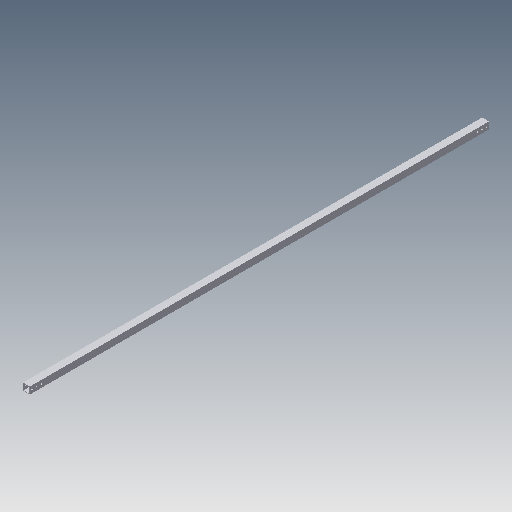
# Autodesk Inventor part: □15
Saved by Autodesk Inventor 2019.4 (Build 234330000, 330)
## iProperties
Created: 2018-08-09
Part Number: □15
Material: 一般
Document SubType Name: Modeling
Designer: Owner
Density: 1 g/cm^3
Appearance: 既定
Mass: 44.7093 g
Surface Area: 896.475 cm^2
Volume: 44.7093 cm^3
Author: Owner
Autodesk Inventor part; units mm, degrees
ref_plane "YZ Plane" through (0, 0, 0) normal (1, 0, 0) x (0, 1, 0)
ref_plane "XZ Plane" through (0, 0, 0) normal (0, 1, 0) x (-1, 0, 0)
ref_plane "XY Plane" through (0, 0, 0) normal (0, 0, 1) x (1, 0, 0)
sketch "スケッチ1" plane through (0, 0, 0) normal (0, 0, 1) x (1, 0, 0)
  line L0 (7.5, 7.5) -> (-7.5, 7.5)
  line L1 (-7.5, 7.5) -> (-7.5, -7.5)
  line L2 (-7.5, -7.5) -> (7.5, -7.5)
  line L3 (7.5, -7.5) -> (7.5, 7.5)
  line L4 (7.5, 7.5) -> (-7.5, -7.5) construction
  line L5 (-7.5, 7.5) -> (7.5, -7.5) construction
  point P0 (0, 0)
  dimension "d0" = 15
  dimension "d1" = 15
  constraints: 12 end point, 2 midpoint, 2 parallel, 1 horizontal, 1 perpendicular
  measures "d0" distance of L2.end L1.end
  measures "d1" distance of L1.end L0.end
extrude "押し出し1" add sketch "スケッチ1" along normal blind 1000
shell "シェル1" thickness 1 removed faces 2 at (-2.5, 2.5, 0) at (-2.5, 2.5, 1000)
sketch "スケッチ2" plane through (-7.5, -7.5, 0) normal (-1, 0, 0) x (0, 0, 1)
  line L0 (0, 0) -> (0, 15) projected
  line L1 (0, 15) -> (1000, 15) projected
  line L2 (1000, 0) -> (1000, 15) projected
  line L3 (0, 0) -> (1000, 0) projected
  line L4 (1000, 15) -> (1000, 0) projected
  line L5 (0, 15) -> (0, 0) projected
  point P0 (5, 7.5)
  point P1 (15, 7.5)
  point P2 (25, 7.5)
  point P3 (995, 7.5)
  point P4 (985, 7.5)
  point P5 (975, 7.5)
  point P6 (1000, 7.5)
  point P7 (0, 7.5)
  dimension "d5" = 10
  dimension "d6" = 10
  dimension "d9" = 10
  dimension "d10" = 10
  dimension "d18" = 5
  dimension "d19" = 5
  constraints: 6 horizontal alignment, 2 midpoint
  measures "d5" distance of point (15, 7.5) point (5, 7.5)
  measures "d6" distance of point (25, 7.5) point (15, 7.5)
  measures "d9" distance of point (985, 7.5) point (995, 7.5)
  measures "d10" distance of point (975, 7.5) point (985, 7.5)
  measures "d18" distance of point (1000, 7.5) point (995, 7.5)
  measures "d19" distance of point (0, 7.5) point (5, 7.5)
hole "穴1" at (-7.5, 0, 5) at (-7.5, 0, 15) at (-7.5, 0, 25) at (-7.5, 0, 995) at (-7.5, 0, 985) at (-7.5, 0, 975) direction (1, 0, 0) diameter 3.2 end through all
equation "\"d6\" = d5"
equation "\"d10\" = d9"
